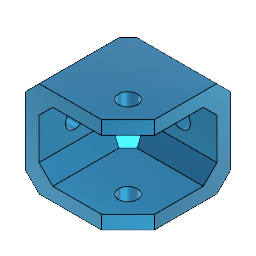
XY Corner Pulley Buddy (Autodesk Fusion 360 design; units mm, degrees)
Autodesk Fusion 360 part; units mm, degrees
note: some values were not read from the file. Set by a fixed rule: which sketch regions a step uses.
sketch "Sketch1" plane through (0, 0, 0) normal (0, 0, 1) x (1, 0, 0)
  line L0 (0, 0) -> (0, -30)
  line L1 (0, -30) -> (4, -30)
  line L2 (4, -30) -> (4, -4)
  line L3 (4, -4) -> (30, -4)
  line L4 (30, -4) -> (30, 0)
  line L5 (30, 0) -> (0, 0)
  circle A0 centre (21, -21) radius 2.75
  line L6 (4, -30) -> (30, -30)
  line L7 (30, -30) -> (30, -4)
  line L8 (12, -30) -> (30, -12) construction
  line L9 (30, -22.253) -> (22.253, -30)
  dimension "d1491" = 4
  dimension "d1509" = 5.5
  dimension "d1510" = 21
  dimension "d1511" = 21
  dimension "d1517" = 45
  dimension "d1539" = 0
  dimension "d1540" = 0
  dimension "d1541" = 0
  dimension "d1542" = 0
  dimension "d1551" = 0
  dimension "d1552" = 0
  dimension "d1553" = 0
  dimension "d1554" = 0
  dimension "d1568" = 0
  dimension "d1569" = 0
  dimension "d1570" = 0
  dimension "d1571" = 0
  dimension "d1580" = 0
  dimension "d1581" = 0
  dimension "d1582" = 0
  dimension "d1583" = 0
  dimension "d1592" = 0
  dimension "d1593" = 0
  dimension "d1594" = 0
  dimension "d1595" = 0
  dimension "d1607" = 0
  dimension "d1608" = 0
  dimension "d1609" = 0
  dimension "d1610" = 0
  dimension "d1663" = 0
  dimension "d1664" = 0
  dimension "d1665" = 0
  dimension "d1666" = 0
  dimension "d1671" = 0
  dimension "d1672" = 0
  dimension "d1673" = 0
  dimension "d1674" = 0
  dimension "d1688" = 0
  dimension "d1689" = 0
  dimension "d1690" = 0
  dimension "d1691" = 0
  dimension "d1696" = 0
  dimension "d1697" = 0
  dimension "d1698" = 0
  dimension "d1699" = 0
  dimension "d1708" = 0
  dimension "d1709" = 0
  dimension "d1710" = 0
  dimension "d1711" = 0
  dimension "d1742" = 0
  dimension "d1743" = 0
  dimension "d1744" = 0
  dimension "d1745" = 0
  dimension "d1774" = 0
  dimension "d1775" = 0
  dimension "d1776" = 0
  dimension "d1777" = 0
  dimension "d1786" = 0
  dimension "d1787" = 0
  dimension "d1788" = 0
  dimension "d1789" = 0
  dimension "d2119" = 0
  dimension "d2120" = 0
  dimension "d2121" = 0
  dimension "d2122" = 0
  dimension "d2864" = 0
  dimension "d2865" = 0
  dimension "d2866" = 0
  dimension "d2867" = 0
  dimension "d2904" = 0
  dimension "d2905" = 0
  dimension "d2906" = 0
  dimension "d2907" = 0
  dimension "d2912" = 0
  dimension "d2913" = 0
  dimension "d2914" = 0
  dimension "d2915" = 0
  dimension "d1" = 30
  dimension "d2" = 30
  dimension "d307" = 4.5
  constraint vertical L0
  constraint perpendicular L0 L1
  constraint perpendicular L1 L2
  constraint perpendicular L2 L3
  constraint perpendicular L3 L4
  constraint perpendicular L0 L5
  constraint equal L1 L4
  constraint equal L0 L5
  constraint coincident L0.start L5.end
  constraint perpendicular L2 L6
  constraint perpendicular L3 L7
  constraint midpoint A0.centre L8
  constraint coincident L7 L8.end
  constraint coincident L7 L9.start
  constraint coincident L6 L9.end
  measures "d1491" horizontal distance of L0.end L1.end
  measures "d1509" diameter of A0
  measures "d1510" horizontal distance of L0.start A0.centre
  measures "d1511" vertical distance of L0.start A0.centre
  measures "d1517" angle of L3 L8
  measures "d1" vertical distance of L0.start L0.end
  measures "d2" horizontal distance of L0.start L4.end
  measures "d307" distance of A0 L9
extrude "Extrude1" add sketch "Sketch1" along normal mid plane 20 contours L0 L1 L2 L3 L4 L5
extrude "Extrude5" add sketch "Sketch1" against normal blind 4 from surface at -10 contours L0 L1 L2 L3 L4 L5 | L2 L3 L6 L7 L9
extrude "Extrude12" add 1 faces at (16.6651, -6.1467, -14) along direction (0, 0, 1) blind 4 from surface at 24
chamfer "Chamfer2" distance 5 angle 45 2 edges at (4, -4, 0) (0, 0, 0)
sketch "Sketch3" plane through (0, -30, 0) normal (0, -1, 0) x (1, 0, 0)
  line L0 (30, 14) -> (5, 14)
  line L1 (5, -14) -> (30, -14)
  line L2 (30, 14) -> (30, -14)
  line L3 (0, 0) -> (-1.5, 0) construction
  line L4 (0, 4.5) -> (-1.5, 3)
  line L5 (-1.5, 3) -> (-1.5, -3)
  line L6 (-1.5, -3) -> (0, -4.5)
  line L7 (0, 14) -> (5, 14)
  line L8 (5, -14) -> (0, -14)
  line L9 (0, -14) -> (0, 14)
  dimension "d3" = 1.5
  dimension "d4" = 6
  constraint coincident L3.start origin
  constraint horizontal L3
  constraint midpoint L3.end L5
  constraint perpendicular L4 L6
  constraint symmetric L3 L4.start L6.end
  measures "d3" distance of L3.start L3.end
  measures "d4" vertical distance of L4.end L5.end
extrude "Extrude15" add sketch "Sketch3" along normal blind 6.5 from surface at -25 contours L4 L5 L6 L9
hole "Hole5" at (4, -19.5, 0) direction (-1, 0, 0) diameter 5.5 depth 10 tip angle 118
sketch "Sketch5" plane through (-1.5, 0, 0) normal (-1, 0, 0) x (0, -1, 0)
  circle A0 centre (19.5, 0) radius 2.75
  line L0 (27, -5) -> (12, -5)
  line L1 (12, -5) -> (12, 5)
  line L2 (12, 5) -> (27, 5)
  line L3 (27, 5) -> (27, -5)
  line L4 (27, -5) -> (12, 5) construction
  line L5 (12, -5) -> (27, 5) construction
  line L6 (30, -14) -> (30, 14)
  point P0 (19.5, 0)
  dimension "d345" = 10
  dimension "d346" = 15
  dimension "d348" = 3
  constraint perpendicular L0 L1
  constraint parallel L0 L2
  constraint parallel L1 L3
  constraint horizontal L0
  constraint coincident L4 P0
  constraint coincident L5 P0
  constraint coincident P0 A0.centre
  measures "d345" distance of L0.end L1.end
  measures "d346" distance of L1.end L2.end
  measures "d348" distance of L2.end L6
chamfer "Chamfer6" distance 1.5 angle 45 1 edges at (-1.5, -5, 0)
ref_plane "WorkPlane1" through (0, 0, 0) normal (-0.707107, -0.707107, 0) x (0, 0, 1)
mirror "Mirror1" about plane through (0, 0, 0) normal (-0.707107, -0.707107, 0) of "Extrude15", "Hole5", "Chamfer6"
chamfer "Chamfer3" distance 4 angle 45 12 edges at (19.5, -4, 10) (4, -19.5, 10) (6.5, -6.5, 10) (19.5, -4, -10) (6.5, -6.5, -10) (4, -19.5, -10) (0, -17.5, 14) (17.5, 0, 14) (17.5, 0, -14) (0, -17.5, -14) (2.5, -2.5, 14) (2.5, -2.5, -14)
equation "d1511 = d1510"
named bodies: "XY Corner Pulley Buddy"
